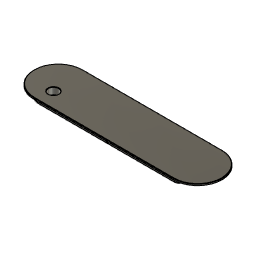
ThroatPlate v3 (Autodesk Fusion 360 design; units mm, degrees)
Autodesk Fusion 360 part; units mm, degrees
sketch "Sketch1" plane through (0, 0, 0) normal (0, 0, 1) x (1, 0, 0)
  line L0 (0, 0) -> (-365.125, 0) construction
  line L1 (-365.125, 0) -> (-365.125, 47.244) construction
  line L2 (-365.125, 47.244) -> (0, 47.244) construction
  line L3 (0, 47.244) -> (0, -47.244) construction
  line L4 (0, -47.244) -> (-365.125, -47.244) construction
  line L5 (-365.125, -47.244) -> (-365.125, 47.244) construction
  line L6 (-47.244, 47.244) -> (-47.244, -47.244) construction
  arc A0 (-47.244, -47.244) -> (-47.244, 47.244) centre (-47.244, 0) ccw
  line L7 (-317.881, 47.244) -> (-317.881, -47.244) construction
  arc A1 (-317.881, 47.244) -> (-317.881, -47.244) centre (-317.881, 0) ccw
  line L8 (-317.881, 47.244) -> (-47.244, 47.244)
  line L9 (-47.244, -47.244) -> (-317.881, -47.244)
  line L10 (-365.125, -47.244) -> (-310.125, -47.244) construction
  line L11 (-310.125, -47.244) -> (-310.125, -17.244) construction
  line L12 (-310.125, -17.244) -> (-365.125, -17.244) construction
  line L13 (-365.125, -17.244) -> (-365.125, -47.244) construction
  circle A2 centre (-310.125, -17.244) radius 10
  dimension "d3" = 365.125
  dimension "d4" = 47.244
  dimension "d5" = 365.125
  dimension "d6" = 94.488
  dimension "d10" = 55
  dimension "d11" = 30
  dimension "d12" = 20
  constraint coincident L0.start origin
  constraint horizontal L0
  constraint perpendicular L0 L1
  constraint horizontal L2
  constraint vertical L3
  constraint horizontal L4
  constraint vertical L5
  constraint coincident L2 L6.start
  constraint coincident L4 L6.end
  constraint perpendicular L4 L6
  constraint midpoint L6 A0.centre
  constraint tangent L3 A0
  constraint coincident L2 L7.start
  constraint coincident L4 L7.end
  constraint perpendicular L4 L7
  constraint midpoint L7 A1.centre
  constraint tangent L5 A1
  constraint horizontal L10
  constraint vertical L11
  constraint horizontal L12
  constraint vertical L13
  constraint coincident L11.end L12.start
  measures "d3" distance of L0.start L0.end
  measures "d4" distance of L0.end L1.end
  measures "d5" distance of L1.end L2.end
  measures "d6" distance of L1.end L4.end
  measures "d10" distance of L4.end L10.end
  measures "d11" distance of L4.end L12.end
  measures "d12" diameter of A2
extrude "Extrude1" add sketch "Sketch1" along normal blind 2.9
sketch "Sketch2" plane through (0, 0, 0) normal (0, 0, -1) x (1, 0, 0)
  circle A0 centre (-310.125, 17.244) radius 10 construction
  arc A1 (-317.881, 47.244) -> (-317.881, -47.244) centre (-317.881, 0) ccw construction
  line L0 (-317.881, -47.244) -> (-47.244, -47.244) construction
  arc A2 (-47.244, -47.244) -> (-47.244, 47.244) centre (-47.244, 0) ccw construction
  line L1 (-47.244, 47.244) -> (-317.881, 47.244) construction
  line L2 (0, 0) -> (-365.125, 0) construction
  line L3 (0, 0) -> (-31, 0) construction
  line L4 (-31, 0) -> (-31, -100) construction
  line L5 (0, 0) -> (-52.5, 0) construction
  line L6 (-52.5, 0) -> (-52.5, -100) construction
  line L7 (-52.5, 0) -> (-44.5, 0) construction
  line L8 (-44.5, 0) -> (-44.5, -100) construction
  line L9 (-52.5, 0) -> (-40, 0) construction
  line L10 (-40, 0) -> (-40, -100) construction
  line L11 (-52.5, -47.244) -> (-52.5, -39.744) construction
  line L12 (-52.5, -39.744) -> (-52.5, -34.144) construction
  line L13 (-52.5, -39.744) -> (-52.5, -29.844) construction
  line L14 (-52.5, -39.744) -> (-52.5, -18.994) construction
  line L15 (-52.5, -39.744) -> (47.5, -39.744) construction
  line L16 (-52.5, -34.144) -> (47.5, -34.144) construction
  line L17 (-52.5, -29.844) -> (47.5, -29.844) construction
  line L18 (-52.5, -18.994) -> (47.5, -18.994) construction
  line L19 (-52.5, -39.744) -> (-317.881, -39.744)
  arc A3 (-52.5, -39.744) -> (-44.5, -34.144) centre (-53.3125, -30.069) ccw
  arc A4 (-40, -29.844) -> (-44.5, -34.144) centre (-36.8886, -37.6048) ccw
  arc A5 (-40, -29.844) -> (-31.5659, -21.0335) centre (-45.5992, -16.0418) ccw
  line L20 (0, 0) -> (-365.125, 0) construction
  arc A6 (-31.5659, 21.0335) -> (-40, 29.844) centre (-45.5992, 16.0418) ccw
  arc A7 (-44.5, 34.144) -> (-40, 29.844) centre (-36.8886, 37.6048) ccw
  arc A8 (-44.5, 34.144) -> (-52.5, 39.744) centre (-53.3125, 30.069) ccw
  line L21 (-52.5, 39.744) -> (-317.881, 39.744)
  line L22 (-31, -18.994) -> (-31, 18.994) construction
  line L23 (-317.881, -47.244) -> (-317.881, -39.744) construction
  line L24 (-365.125, 0) -> (-352.125, 0) construction
  arc A9 (-317.881, 39.744) -> (-317.881, -39.744) centre (-311.9393, 0) ccw
  line L25 (0, 0) -> (-13, 0) construction
  arc A10 (-28.8515, -18.7555) -> (-28.8515, 18.7555) centre (-32.0214, 0) ccw
  arc A11 (-28.8515, -18.7555) -> (-31.5659, -21.0335) centre (-28.2683, -22.2065) ccw
  arc A12 (-31.5659, 21.0335) -> (-28.8515, 18.7555) centre (-28.2683, 22.2065) ccw
  circle A13 centre (-310.125, 17.244) radius 10
  dimension "d22" = 31
  dimension "d23" = 52.5
  dimension "d24" = 100
  dimension "d25" = 100
  dimension "d26" = 8
  dimension "d27" = 100
  dimension "d28" = 12.5
  dimension "d29" = 100
  dimension "d34" = 7.5
  dimension "d35" = 5.6
  dimension "d36" = 9.9
  dimension "d37" = 20.75
  dimension "d38" = 100
  dimension "d39" = 100
  dimension "d40" = 100
  dimension "d41" = 100
  dimension "d42" = 7.5
  dimension "d43" = 13
  dimension "d44" = 13
  dimension "d45" = 3.5
  constraint coincident L2.start L3.start
  constraint coincident L2 L3.end
  constraint perpendicular L2 L4
  constraint coincident L2 L5.end
  constraint perpendicular L2 L6
  constraint perpendicular L2 L8
  constraint coincident L2 L9.end
  constraint perpendicular L9 L10
  constraint coincident L0 L11.start
  constraint coincident L6 L11.start
  constraint perpendicular L0 L11
  constraint perpendicular L0 L12
  constraint coincident L6 L13.end
  constraint parallel L6 L14
  constraint perpendicular L4 L15
  constraint horizontal L16
  constraint horizontal L17
  constraint perpendicular L6 L18
  constraint perpendicular L12 L19
  constraint coincident L8 A3.end
  constraint coincident L16 A3.end
  constraint coincident L10 A4.start
  constraint coincident L17 A4.start
  constraint coincident L18 L22.start
  constraint coincident L4 L22.start
  constraint symmetric L11.end L20 A8.end
  constraint symmetric L19.end L20 L21.end
  constraint symmetric A3.end L20 A7.start
  constraint symmetric A3 L20 A8
  constraint symmetric A4.start L20 A6.end
  constraint symmetric A4 L20 A7
  constraint symmetric L22.start L20 L22.end
  constraint symmetric A5 L20 A6
  constraint coincident A1.end L0.start
  constraint perpendicular L0 L23
  constraint coincident L19.end L23.end
  constraint coincident L2.end L20.end
  constraint parallel L20 L24
  constraint coincident L24.end A9
  constraint coincident L5 L25.end
  constraint coincident L25.end A10
  constraint coincident L22.start A10
  constraint tangent A10 A11
  constraint tangent A5 A11
  constraint coincident L22.end A10
  constraint coincident L22.end A6
  constraint tangent A10 A12
  constraint tangent A6 A12
  constraint equal A11 A12
  measures "d22" distance of L2.start L3.end
  measures "d23" distance of L2.start L5.end
  measures "d24" distance of L5.end L6.end
  measures "d25" distance of L3.end L4.end
  measures "d26" distance of L5.end L7.end
  measures "d27" distance of L7.end L8.end
  measures "d28" distance of L5.end L9.end
  measures "d29" distance of L9.end L10.end
  measures "d34" distance of L11.start L11.end
  measures "d35" distance of L11.end L12.end
  measures "d36" distance of L11.end L13.end
  measures "d37" distance of L11.end L14.end
  measures "d38" distance of L11.end L15.end
  measures "d39" distance of L12.end L16.end
  measures "d40" distance of L13.end L17.end
  measures "d41" distance of L14.end L18.end
  measures "d42" distance of A1.end L19.end
  measures "d43" distance of L2.end L24.end
  measures "d44" distance of L2.start L25.end
  measures "d45" radius of A11
extrude "Extrude2" add sketch "Sketch2" along normal blind 11
chamfer "Chamfer1" distance 0.7 angle 45 5 edges at (-182.5625, 47.244, 2.9) (-365.125, 0, 2.9) (-182.5625, -47.244, 2.9) (0, 0, 2.9) (-319.4483, -13.6278, 2.9)
chamfer "Chamfer1" distance 0.7 angle 45 13 edges at (-185.1905, -39.744, -11) (-352.125, 0, -11) (-47.7447, -38.023, -11) (-42.665, -31.5597, -11) (-34.8398, -26.3416, -11) (-34.8398, 26.3416, -11) (-30.5183, 19.5256, -11) (-13, 0, -11) (-30.5183, -19.5256, -11) (-42.665, 31.5597, -11) (-47.7447, 38.023, -11) (-185.1905, 39.744, -11) (-319.4483, -20.8602, -11)
sketch "Sketch3" plane through (0, -39.744, 0) normal (0, -1, 0) x (1, 0, 0)
  line L0 (-317.881, -10.3) -> (-52.5, -10.3)
  line L1 (-52.5, -10.3) -> (-52.5, 0)
  line L2 (-52.5, 0) -> (-317.881, 0)
  line L3 (-317.881, 0) -> (-317.881, -10.3)
  line L4 (-44.5, 0) -> (-40, 0)
  line L5 (-31.5659, 0) -> (-40, 0)
  line L6 (-31.5659, 0) -> (-28.8515, 0)
  line L7 (-13, 0) -> (-28.8515, 0)
  line L8 (-31.5659, 0) -> (-28.8515, 0)
  line L9 (-31.5659, 0) -> (-40, 0)
  line L10 (-44.5, 0) -> (-40, 0)
  line L11 (-44.5, 0) -> (-52.5, 0)
  line L12 (-52.5, 0) -> (-317.881, 0)
  line L13 (-317.881, 0) -> (-352.125, 0)
  line L14 (-317.881, 0) -> (-52.5, 0)
  line L15 (-44.5, 0) -> (-52.5, 0)
  line L16 (-317.881, 0) -> (-365.125, 0)
  line L17 (-317.881, 0) -> (-47.244, 0)
  line L18 (0, 0) -> (-47.244, 0)
  line L19 (-47.244, 0) -> (-317.881, 0)
  line L20 (-182.5625, 0) -> (-182.5625, -10.3) construction
  line L21 (-182.5625, 0) -> (-182.5625, -5.15) construction
  constraint midpoint L19 L20.start
  constraint coincident L0 L20.end
  constraint perpendicular L0 L20
  constraint midpoint L20 L21.end
hole "Hole1" at (-182.5625, -39.744, -5.15) direction (0, 1, 0) diameter 3.2 depth 20 tip angle 118 countersink diameter 8.5 countersink angle 90
ref_plane "WorkPlane1" through (-352.125, 0, 0) normal (1, 0, 0) x (0, 1, 0)
sketch "Sketch4" plane through (-352.125, 0, 0) normal (1, 0, 0) x (0, 1, 0)
  line L0 (39.044, -11) -> (-39.044, -11)
  line L1 (-39.744, 0) -> (39.744, 0)
  line L2 (0, 0) -> (0, -11)
  line L3 (0, 0) -> (0, -5.5)
  constraint coincident L2.start L3.start
  constraint midpoint L0 L2.end
  constraint midpoint L2 L3.end
hole "Hole2" at (-352.125, 0, -5.6194) direction (1, 0, 0) diameter 3.2 depth 20 tip angle 118 countersink diameter 8.5 countersink angle 90
equation "TopL = ( ( 14 + ( 3 / 8 ) ) * 25.4 ) * 1 mm" comment "Overall Length"
equation "TopW = ( 3.72 * 25.4 ) * 1 mm" comment "Overall Width"
equation "d3 = TopL"
equation "d4 = TopW / 2"
equation "d5 = TopL"
equation "d6 = TopW"
equation "HoleB = 30 mm" comment "Hole from Bottom"
equation "HoleR = 55 mm" comment "Hole From Right"
equation "HoleD = 20 mm" comment "Hole Diameter"
equation "TopT = 2.9 mm" comment "Top Thickness"
equation "d14 = TopT"
equation "TrailEndO = 13 mm" comment "Offset on left"
equation "TrailFC = 52.5 mm" comment "Beginning of first curve"
equation "TrailSC = 8 mm" comment "Beginning of Second Curve"
equation "TrailTC = 12.5 mm" comment "Beginning of Thrid Curve"
equation "TrailFlat = 31 mm"
equation "d22 = TrailFlat"
equation "d23 = TrailFC"
equation "d26 = TrailSC"
equation "d28 = TrailTC"
equation "TrailFW = 5.6 mm" comment "First Curve Width"
equation "TrailSW = 9.9 mm" comment "Second Curve Width"
equation "TrailTW = 20.75 mm" comment "Third Cure Width"
equation "BottomWO = 7.5 mm" comment "Bottom Width Offset"
equation "d34 = BottomWO"
equation "d35 = TrailFW"
equation "d36 = TrailSW"
equation "d37 = TrailTW"
equation "d42 = BottomWO"
equation "d43 = TrailEndO"
equation "d44 = TrailEndO"
equation "BottomT = 11 mm" comment "BottomThickness"
equation "d47 = BottomT"
equation "d55 = -TopL + TrailEndO"
